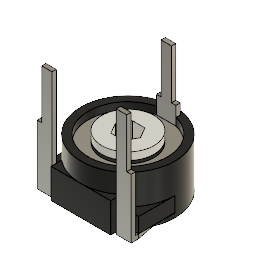
Finger iteration (Autodesk Fusion 360 archive; units mm, degrees)
design "Piher Potentiometer PT-6MH103A20202E"
Autodesk Fusion 360 part; units mm, degrees
note: some values were not read from the file. Set by a fixed rule: which sketch regions a step uses.
sketch "Sketch1" plane through (0, 0, 0) normal (0, 0, 1) x (1, 0, 0)
  circle A0 centre (0, 0) radius 3.15
  circle A1 centre (0, 0) radius 1.15
  line L0 (-0.4186, 0.725) -> (-0.8372, 0)
  line L1 (-0.8372, 0) -> (-0.4186, -0.725)
  line L2 (-0.4186, -0.725) -> (0.4186, -0.725)
  line L3 (0.4186, -0.725) -> (0.8372, 0)
  line L4 (0.8372, 0) -> (0.4186, 0.725)
  line L5 (0.4186, 0.725) -> (-0.4186, 0.725)
  line L6 (-3.15, 0) -> (3.15, 0) construction
  line L7 (0, 3.15) -> (0, -3.15) construction
  line L8 (-2.5, -1) -> (-2.5, -2.9336) construction
  line L9 (2.5, -1) -> (2.5, -2.9336) construction
  line L10 (0, -3.15) -> (0, -2.9336) construction
  line L11 (-2.5, -2.9336) -> (2.5, -2.9336) construction
  line L12 (2.5, -1) -> (-2.5, -1) construction
  line L13 (-2.5, -1) -> (-2.5, -1.5484)
  line L14 (-2.85, -2.9336) -> (-3.15, -2.9336)
  line L15 (-3.15, -2.9336) -> (-3.15, 0)
  circle A2 centre (0, 0) radius 1.75
  circle A3 centre (0, 0) radius 2.65
  line L16 (2.15, -1) -> (2.15, -2.9336)
  line L17 (2.85, -2.9336) -> (2.85, -1)
  line L18 (2.85, -1) -> (2.15, -1)
  line L19 (3.15, -2.9336) -> (3.15, 0)
  line L20 (2.85, -2.9336) -> (3.15, -2.9336)
  line L21 (2.15, -2.9336) -> (2.85, -2.9336)
  line L22 (-2, -3.15) -> (2, -3.15)
  line L23 (2, -3.15) -> (2, -2.4336)
  line L24 (-2, -3.15) -> (-2, -3.0261)
  line L25 (-2, -3.0261) -> (-2, -2.4336)
  line L26 (-2, -2.4336) -> (-3.15, -2.4336)
  line L27 (2, -2.4336) -> (3.15, -2.4336)
  line L28 (-0.65, 2.8664) -> (0.65, 2.8664)
  line L29 (0.65, 2.8664) -> (0.65, 2.5664)
  line L30 (0.65, 2.5664) -> (-0.65, 2.5664)
  line L31 (-0.65, 2.5664) -> (-0.65, 2.8664)
  line L32 (-0.35, 2.8664) -> (-0.35, 2.5664)
  line L33 (0.35, 2.8664) -> (0.35, 2.5664)
  line L34 (2.15, -2.6336) -> (3.15, -2.6336)
  line L35 (2.85, -1) -> (3.15, -2.4336)
  line L36 (-2.15, -1) -> (-2.15, -2.9336)
  line L37 (-2.85, -2.9336) -> (-2.85, -1)
  line L38 (-2.15, -2.9336) -> (-2.85, -2.9336)
  line L39 (-2.15, -2.6336) -> (-3.15, -2.6336)
  line L40 (-2.85, -1) -> (-3.15, -2.4336)
  line L41 (-2.85, -1) -> (-2.15, -1)
  dimension "d1" = 6.3
  dimension "d2" = 2.3
  dimension "d3" = 1.45
  dimension "d7" = 1
  dimension "d8" = 5
  dimension "d17" = 3.5
  dimension "d18" = 0.5
  dimension "d19" = 4
  dimension "d55" = 1.3
  dimension "d56" = 0.3
  dimension "d57" = 0.7
  dimension "d58" = 0.5
  dimension "d59" = 0.3
  dimension "d61" = 0.7
  dimension "d62" = 0.3
  dimension "d63" = 5.8
  constraint coincident A0.centre A1.centre
  constraint horizontal L5
  constraint coincident A0 L6.start
  constraint coincident A0 L6.end
  constraint horizontal L6
  constraint coincident A0.centre L6
  constraint coincident A0 L7.start
  constraint vertical L7
  constraint coincident A0 L7.end
  constraint coincident A0.centre L7
  constraint vertical L8
  constraint vertical L9
  constraint horizontal L11
  constraint vertical L10
  constraint coincident L10.end L11
  constraint horizontal L12
  constraint symmetric L7 L8 L9
  constraint coincident L8 L13.end
  constraint perpendicular L12 L13
  constraint concentric A0 A2
  constraint symmetric L10 L14.start L17.start
  constraint symmetric L10 L14.end L19.start
  constraint symmetric L10 L6.start L6.end
  constraint coincident A0 L23.end
  constraint perpendicular L22 L23
  constraint perpendicular L22 L24
  constraint coincident A0 L25.end
  constraint perpendicular L22 L25
  constraint midpoint L7.end L22
  constraint coincident L6.start L15.end
  constraint coincident L15 L26.end
  constraint perpendicular L15 L26
  constraint coincident L19 L27.end
  constraint perpendicular L19 L27
  constraint horizontal L28
  constraint vertical L29
  constraint horizontal L30
  constraint vertical L31
  constraint symmetric L7 L29 L31
  constraint coincident L28 L32.start
  constraint coincident L30 L32.end
  constraint perpendicular L30 L32
  constraint coincident L28 L33.start
  constraint coincident L30 L33.end
  constraint perpendicular L30 L33
  constraint symmetric L7 L32 L33
  constraint horizontal L22
  constraint horizontal L26
  constraint horizontal L20
  constraint coincident L17.start L20.start
  constraint coincident L19 L34.end
  constraint perpendicular L19 L34
  constraint collinear L11 L21
  constraint vertical L17
  constraint horizontal L18
  constraint vertical L16
  constraint collinear L12 L18
  constraint symmetric L7 L16.start L36.start
  constraint symmetric L7 L16.end L36.end
  constraint symmetric L7 L17.start L14.start
  constraint symmetric L7 L17.end L37.end
  constraint symmetric L7 L27.end L26.end
  constraint symmetric L7 L34.start L39.start
  constraint symmetric L7 L34.end L39.end
  constraint coincident L16 L34.start
  measures "d1" diameter of A0
  measures "d2" diameter of A1
  measures "d3" distance of L2 L5
  measures "d7" distance of L6 L12
  measures "d8" distance of L8 L9
  measures "d17" diameter of A2
  measures "d18" distance of A0 A3
  measures "d19" distance of L22.start L22.end
  measures "d55" distance of L28.start L28.end
  measures "d56" distance of L28.end L29.end
  measures "d57" distance of L32 L33
  measures "d58" distance of L11 L26
  measures "d59" distance of L21 L34
  measures "d61" distance of L16 L17
  measures "d62" distance of L17 L19
  measures "d63" distance of L11 L28
extrude "Extrude1" add sketch "Sketch1" along normal blind 3.3 contours A0 A3 L18 L28 L29 L31 L35 L40 L41 | A0 L17 L35 | A0 L37 L40 | A0 A3 L16 L17 L18 | A0 A3 L36 L37 L41 | A0 A3 L16 L36 | A3 L16 L18 L29 L30 L31 L36 L41 | A3 L16 L18 | A3 L36 L41 | A3 L29 L30 L33 | A3 L28 L29 L33 | A3 L28 L31 L32 | A3 L30 L31 L32 | A3 L30 L32 L33 | A3 L28 L32 L33 | A2 makes body 1 in component "Base"
extrude "Extrude2" cut sketch "Sketch1" against normal blind 0.5 from surface at 3.3 contours A3 L16 L18 L29 L30 L31 L36 L41 | A3 L16 L18 | A3 L36 L41 | A3 L29 L30 L33 | A3 L30 L31 L32 | A3 L30 L32 L33 | A2 bodies 1 in component "Base"
extrude "Extrude4" add sketch "Sketch1" along normal blind 2 contours A0 L22 L23 | A0 L22 L24 L25 bodies 1 in component "Base"
extrude "Extrude1'" add sketch "Sketch1" along normal blind 3.5 separate body contours A1 makes body 2 in component "Rotor"
extrude "Extrude2'" add sketch "Sketch1" against normal blind 0.5 from surface at 3.5 contours A2 bodies 2 in component "Rotor"
extrude "Extrude1''" add sketch "Sketch1" along normal blind 0.3 separate body contours A0 L17 L27 L35 | A0 L17 L35 | L17 L19 L27 L34 | A0 L37 L40 | A0 L26 L37 L40 | L15 L26 L37 L39 | A0 L16 L17 L27 | A0 A3 L16 L17 L18 | L17 L19 L20 L34 | L16 L17 L27 L34 | A0 A3 L36 L37 L41 | A0 L26 L36 L37 | L14 L15 L37 L39 | L26 L36 L37 L39 | A3 L16 L18 | L16 L17 L21 L34 | L36 L37 L38 L39 | A3 L36 L41 makes body 3 at (-2.4833, -2.1224, 0) makes body 4 at (2.4833, -2.1224, 0.3) in component "Prongs"
extrude "Extrude2''" add sketch "Sketch1" along normal blind 0.3 from surface at 2.5 separate body contours A3 L16 L18 | A3 L16 L18 L30 L36 L41 | A3 L36 L41 | A3 L30 L33 | A3 L28 L29 L33 | A3 L28 L31 L32 | A3 L30 L32 | A3 L30 L32 L33 | A3 L28 L32 L33 makes body 5 in component "Prongs"
extrude "Extrude3" add sketch "Sketch1" along normal blind 4 contours L17 L19 L20 L34 | L14 L15 L37 L39 | L16 L17 L21 L34 | L36 L37 L38 L39 bodies 3 4 in component "Prongs"
extrude "Extrude4'" add sketch "Sketch1" along normal up to surface (1.2 mm away) from surface at 2.8 contours A3 L29 L30 L33 | A3 L28 L29 L33 | A3 L28 L31 L32 | A3 L30 L31 L32 | A3 L30 L32 L33 | A3 L28 L32 L33 bodies 5 in component "Prongs"
extrude "Extrude5" add sketch "Sketch1" along normal blind 3.3 from surface at 4 contours L16 L17 L21 L34 | L36 L37 L38 L39 | A3 L30 L32 L33 | A3 L28 L32 L33 bodies 3 4 5 in component "Prongs"
combine "Combine1" operation cut target body 1 tool bodies 5 3 4 keep tools in component "Base"
extrude "Extrude5'" add sketch "Sketch1" along normal blind 1 from surface at 0.3 contours A0 L19 L35 | A0 L15 L40 | A0 L17 L27 L35 | A0 L26 L37 L40 | A0 L16 L17 L27 | A0 L26 L36 L37 | A0 L16 L27 | A0 L26 L36 bodies 1 in component "Base"
component "Base" placed x (1, 0, 0) y (0, 1, 0) z (0, 0, 1) at (0, 0, 0)
component "Rotor" placed x (1, 0, 0) y (0, 1, 0) z (0, 0, 1) at (0, 0, 0)
component "Prongs" placed x (1, 0, 0) y (0, 1, 0) z (0, 0, 1) at (0, 0, 0)
